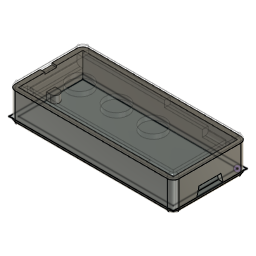
RPI-Shortcut-Keyboard-Case v9 (Autodesk Fusion 360 design; units mm, degrees)
Autodesk Fusion 360 part; units mm, degrees
sketch "Sketch1" plane through (0, 0, 0) normal (0, 0, 1) x (1, 0, 0) in component "bottom"
  line L0 (0, 0) -> (-53, 0)
  line L1 (-53, 0) -> (-53, -22)
  line L2 (-53, -22) -> (0, -22)
  line L3 (0, -22) -> (0, 0)
  line L4 (1.6, 1.6) -> (-54.6, 1.6)
  line L5 (-54.6, 1.6) -> (-54.6, -23.6)
  line L6 (-54.6, -23.6) -> (1.6, -23.6)
  line L7 (1.6, -23.6) -> (1.6, 1.6)
  dimension "d1" = 53
  dimension "d2" = 22
  dimension "d3" = 1.6
  constraint horizontal L0
  constraint vertical L1
  constraint horizontal L2
  constraint vertical L3
  constraint coincident L0.start L3.end
  measures "d1" distance of L0.start L0.end
  measures "d2" distance of L0.start L2.end
extrude "Extrude1" add sketch "Sketch1" against normal blind 1.6 contours L0 L1 L2 L3 | L4 L5 L6 L7 makes body 1 in component "bottom"
extrude "Extrude2" add sketch "Sketch1" along normal blind 8.6 bodies 1 in component "bottom"
sketch "Sketch3" plane through (0, 0, 0) normal (0, 0, 1) x (1, 0, 0) in component "bottom"
  line L0 (0, 0) -> (-1.5, 0) construction
  line L1 (-1.5, 0) -> (-1.5, -1.5) construction
  line L2 (-1.5, -1.5) -> (0, -1.5) construction
  line L3 (0, -1.5) -> (0, 0) construction
  line L4 (0, -22) -> (-1.5, -22) construction
  line L5 (-1.5, -22) -> (-1.5, -20.5) construction
  line L6 (-1.5, -20.5) -> (0, -20.5) construction
  line L7 (0, -20.5) -> (0, -22) construction
  line L8 (-53, 0) -> (-51.5, 0) construction
  line L9 (-51.5, 0) -> (-51.5, -22) construction
  line L10 (-51.5, -22) -> (-53, -22) construction
  line L11 (-51.5, -9.5) -> (-53, -9.5)
  line L12 (-51.5, -12.5) -> (-53, -12.5)
  line L13 (-3, 0) -> (-3, -1.5)
  line L14 (0, -3) -> (-1.5, -3)
  line L15 (0, -19) -> (-1.5, -19)
  line L16 (-3, -22.0018) -> (-3, -20.5)
  arc A0 (-1.5, -19) -> (-3, -20.5) centre (-1.5, -20.5) ccw
  line L17 (0, -22) -> (-53, -22)
  line L18 (-53, -22) -> (-53, 0)
  line L19 (-53, 0) -> (0, 0)
  line L20 (0, 0) -> (0, -22)
  arc A1 (-51.5, -12.5) -> (-51.5, -9.5) centre (-51.5, -11) ccw
  line L21 (-53, -22) -> (-53, -11) construction
  line L22 (-53, -9.5) -> (-53, 0) construction
  arc A2 (-3, -1.5) -> (-1.5, -3) centre (-1.5, -1.5) ccw
  dimension "d15" = 1.5
  dimension "d16" = 1.5
  dimension "d17" = 3
  dimension "d18" = 1.5
  dimension "d19" = 1.5
  dimension "d20" = 3
  dimension "d21" = 1.5
  dimension "d22" = 22
  dimension "d23" = 3
  constraint horizontal L0
  constraint vertical L1
  constraint horizontal L2
  constraint vertical L3
  constraint coincident L0.start L3.end
  constraint coincident L1.end L2.start
  constraint horizontal L4
  constraint vertical L5
  constraint horizontal L6
  constraint vertical L7
  constraint coincident L5.end L6.start
  constraint horizontal L8
  constraint vertical L9
  constraint horizontal L10
  constraint vertical L21
  constraint midpoint L9 A1.centre
  constraint coincident L9 L11.start
  constraint coincident L11.end L21
  constraint tangent L11 A1
  constraint coincident L9 L12.start
  constraint tangent L12 A1
  constraint tangent L13 A2
  constraint tangent L14 A2
  constraint tangent L15 A0
  constraint tangent L16 A0
  constraint vertical L16
  constraint horizontal L17
  constraint vertical L18
  constraint horizontal L19
  constraint vertical L20
  constraint collinear L21 L22
  measures "d15" distance of L0.start L0.end
  measures "d16" distance of L0.start L2.end
  measures "d17" diameter of A2
  measures "d18" distance of L4.start L4.end
  measures "d19" distance of L4.start L6.end
  measures "d20" diameter of A0
  measures "d21" distance of L8.start L8.end
  measures "d22" distance of L8.start L10.end
  measures "d23" diameter of A1
extrude "Extrude4" add sketch "Sketch3" along normal blind 2.5 contours L11 L12 L18 A1 | L13 L14 L19 L20 A2 | L15 L16 A0 L17 L20 bodies 1 in component "bottom"
sketch "Sketch1 (2)" plane through (0, 0, 8.6) normal (0, 0, 1) x (-1, 0, 0) in component "top"
  line L0 (0, 0) -> (0, 22)
  line L1 (0, 22) -> (53, 22)
  line L2 (53, 22) -> (53, 0)
  line L3 (53, 0) -> (0, 0)
  line L4 (-1.6, 23.6) -> (-1.6, -1.6)
  line L5 (-1.6, -1.6) -> (54.6, -1.6)
  line L6 (54.6, -1.6) -> (54.6, 23.6)
  line L7 (54.6, 23.6) -> (-1.6, 23.6)
  line L8 (-1.6, -1.6) -> (54.6, -1.6)
  line L9 (-1.6, 23.6) -> (-1.6, -1.6)
  line L10 (54.6, 23.6) -> (-1.6, 23.6)
  line L11 (53, 2) -> (2, 2)
  line L12 (2, 2) -> (2, 20)
  line L13 (2, 20) -> (51, 20)
  line L14 (51, 20) -> (51, 2)
  line L15 (0, 22) -> (10, 22) construction
  line L16 (10, 22) -> (10, 0)
  line L17 (53, 22) -> (50, 22) construction
  line L18 (50, 22) -> (50, 19) construction
  line L19 (50, 19) -> (53, 19) construction
  line L20 (53, 19) -> (53, 22) construction
  line L21 (53, 19) -> (51, 19)
  line L22 (51, 2) -> (51, 0)
  line L23 (53, 0) -> (23, 0) construction
  line L24 (23, 0) -> (23, 2)
  dimension "d29" = 10
  dimension "d30" = 3
  dimension "d31" = 3
  dimension "d77" = 30
  constraint horizontal L15
  constraint coincident L0.end L1.start
  constraint coincident L3 L16.end
  constraint perpendicular L3 L16
  constraint horizontal L17
  constraint vertical L18
  constraint horizontal L19
  constraint vertical L20
  constraint coincident L1.end L2.start
  constraint coincident L14 L21.end
  constraint coincident L19 L21.end
  constraint coincident L3 L22.end
  constraint perpendicular L3 L22
  constraint horizontal L23
  constraint coincident L2.end L3.start
  constraint coincident L11 L24.end
  constraint perpendicular L11 L24
  constraint coincident L2 L11.start
  constraint coincident L14.end L11
  measures "d29" distance of L0.end L15.end
  measures "d30" distance of L1.end L17.end
  measures "d31" distance of L1.end L19.end
  measures "d77" distance of L2.end L23.end
extrude "Extrude1'" add sketch "Sketch1 (2)" along normal blind 1.6 separate body contours L0 L1 L3 L11 L12 L13 L16 | L3 L11 L16 L24 | L1 L2 L13 L14 L16 L21 | L3 L11 L22 L24 | L11 L13 L14 L16 | L11 L12 L13 L16 | L2 L3 L11 L22 | L2 L11 L14 L21 | L4 L5 L6 L7 L8 L9 L10 makes body 2 in component "top"
extrude "Extrude2'" add sketch "Sketch1 (2)" against normal blind 3.3 contours L0 L1 L3 L11 L12 L13 L16 | L2 L11 L14 L21 bodies 2 in component "top"
extrude "Extrude3" add sketch "Sketch1 (2)" against normal blind 1 contours L3 L11 L16 L24 | L1 L2 L13 L14 L16 L21 bodies 2 in component "top"
extrude "Extrude7" cut sketch "Sketch1 (2)" along normal blind 1.2 contours L3 L11 L22 L24 bodies 2 in component "top"
sketch "Sketch2" plane through (0, 0, 10.2) normal (0, 0, 1) x (-1, 0, 0) in component "top"
  line L0 (54.6, 23.6) -> (-1.6, 23.6)
  line L1 (-1.6, 23.6) -> (-1.6, -1.6)
  line L2 (-1.6, -1.6) -> (54.6, -1.6)
  line L3 (54.6, -1.6) -> (54.6, 23.6)
  line L4 (53, 0) -> (46, 0) construction
  line L5 (46, 0) -> (46, 8) construction
  line L6 (46, 8) -> (53, 8) construction
  line L7 (53, 8) -> (53, 0) construction
  line L8 (46, 8) -> (42.5, 8) construction
  line L9 (42.5, 8) -> (42.5, 11.5) construction
  line L10 (42.5, 11.5) -> (46, 11.5) construction
  line L11 (46, 11.5) -> (46, 8) construction
  circle A0 centre (42.5, 11.5) radius 4
  circle A1 centre (29.9, 11.5) radius 4
  circle A2 centre (17.3, 11.5) radius 4
  dimension "d36" = 7
  dimension "d37" = 8
  dimension "d38" = 3.5
  dimension "d39" = 3.5
  dimension "d40" = 8
  dimension "d43" = -25.2
  dimension "d44" = 0
  constraint horizontal L4
  constraint vertical L5
  constraint horizontal L6
  constraint vertical L7
  constraint horizontal L8
  constraint vertical L9
  constraint horizontal L10
  constraint vertical L11
  constraint coincident L9.end L10.start
  measures "d36" distance of L4.start L4.end
  measures "d37" distance of L4.start L6.end
  measures "d38" distance of L5.end L8.end
  measures "d39" distance of L5.end L10.end
  measures "d40" diameter of A0
extrude "Extrude4'" cut sketch "Sketch2" against normal blind 2 contours A0 | A1 | A2 bodies 2 in component "top"
fillet "Fillet1" radius 2 4 edges at (1.6, -23.6, 9.4) (1.6, 1.6, 9.4) (-54.6, 1.6, 9.4) (-54.6, -23.6, 9.4) on bodies 2 in component "top"
fillet "Fillet2" radius 1 8 edges at (-54.0142, 1.0142, 10.2) (-54.6, -11, 10.2) (-54.0142, -23.0142, 10.2) (-26.5, -23.6, 10.2) (1.0142, -23.0142, 10.2) (1.6, -11, 10.2) (1.0142, 1.0142, 10.2) (-26.5, 1.6, 10.2) on bodies 2 in component "top"
fillet "Fillet3" radius 1 3 edges at (0, -22, 6.95) (-53, -22, 8.1) (0, 0, 6.95) on bodies 2 in component "top"
fillet "Fillet3" radius 1 2 edges at (-53, -10.5, 5.3) (0, -11, 5.3) on bodies 2 in component "top"
fillet "Fillet3" radius 1 2 edges at (-5, 0, 5.3) (-5, -22, 5.3) on bodies 2 in component "top"
sketch "Sketch5" plane through (1.6, 0, 0) normal (1, 0, 0) x (0, 1, 0) in component "bottom"
  line L0 (-23.6, 8.6) -> (-23.6, -1.6)
  line L1 (-23.6, -1.6) -> (1.6, -1.6)
  line L2 (1.6, -1.6) -> (1.6, 8.6)
  line L3 (1.6, 8.6) -> (-23.6, 8.6)
  line L4 (-11, 8.6) -> (-11, 0) construction
  line L5 (-11, 0) -> (-6.5, 0)
  line L6 (-11, 0) -> (-15.5, 0)
  line L7 (-11, 0) -> (-11, 3) construction
  line L8 (-11, 3) -> (-7.25, 3)
  line L9 (-11, 3) -> (-14.75, 3)
  line L10 (-14.75, 3) -> (-15.5, 0)
  line L11 (-7.25, 3) -> (-6.5, 0)
  dimension "d69" = 4.5
  dimension "d70" = 4.5
  dimension "d71" = 3
  dimension "d72" = 90
  dimension "d73" = 3.75
  dimension "d74" = 3.75
  constraint midpoint L3 L4.start
  constraint perpendicular L3 L4
  constraint perpendicular L4 L5
  constraint perpendicular L4 L6
  constraint perpendicular L5 L7
  constraint perpendicular L4 L9
  measures "d69" distance of L4.end L5.end
  measures "d70" distance of L4.end L6.end
  measures "d71" distance of L4.end L7.end
  measures "d72" angle of L7 L8
  measures "d73" distance of L7.end L8.end
  measures "d74" distance of L7.end L9.end
extrude "Extrude6" cut sketch "Sketch5" against normal blind 1.6 contours L5 L6 L8 L9 L10 L11 bodies 1 in component "bottom"
fillet "Fillet1'" radius 2 4 edges at (1.6, 1.6, 3.5) (1.6, -23.6, 3.5) (-54.6, 1.6, 3.5) (-54.6, -23.6, 3.5) on bodies 1 in component "bottom"
fillet "Fillet2'" radius 1 8 edges at (-54.0142, 1.0142, -1.6) (-26.5, 1.6, -1.6) (1.0142, 1.0142, -1.6) (1.6, -11, -1.6) (1.0142, -23.0142, -1.6) (-26.5, -23.6, -1.6) (-54.0142, -23.0142, -1.6) (-54.6, -11, -1.6) on bodies 1 in component "bottom"
sketch "Sketch4" plane through (-54.6, 0, 0) normal (-1, 0, 0) x (0, -1, 0) in component "bottom"
  line L0 (0.4, -0.6) -> (21.6, -0.6)
  line L1 (21.6, -0.6) -> (21.6, 8.6)
  line L2 (21.6, 8.6) -> (0.4, 8.6)
  line L3 (0.4, 8.6) -> (0.4, -0.6)
  line L4 (11, 8.6) -> (11, 0) construction
  line L5 (11, 8.6) -> (9, 8.6) construction
  line L6 (9, 8.6) -> (9, 8) construction
  line L7 (9, 8) -> (11, 8) construction
  line L8 (11, 8) -> (11, 8.6) construction
  line L9 (9, 8) -> (13, 8)
  line L10 (13, 8) -> (13, 8.6)
  line L11 (13, 8.6) -> (9, 8.6)
  line L12 (9, 8.6) -> (9, 8)
  dimension "d63" = 2
  dimension "d64" = 0.6
  dimension "d65" = 4
  dimension "d66" = 0.6
  constraint midpoint L2 L4.start
  constraint perpendicular L2 L4
  constraint horizontal L5
  constraint vertical L6
  constraint horizontal L7
  constraint vertical L8
  constraint horizontal L9
  constraint vertical L10
  constraint horizontal L11
  constraint vertical L12
  measures "d63" distance of L4.start L5.end
  measures "d64" distance of L4.start L7.end
  measures "d65" distance of L6.end L9.end
  measures "d66" distance of L6.end L5.end
extrude "Extrude5" cut sketch "Sketch4" against normal blind 1.6 contours L2 L9 L10 L11 L12 bodies 1 in component "bottom"
component "bottom" placed x (1, 0, 0) y (0, 1, 0) z (0, 0, 1) at (0, 0, 0)
component "top" placed x (1, 0, 0) y (0, 1, 0) z (0, 0, 1) at (0, 0, 0)
